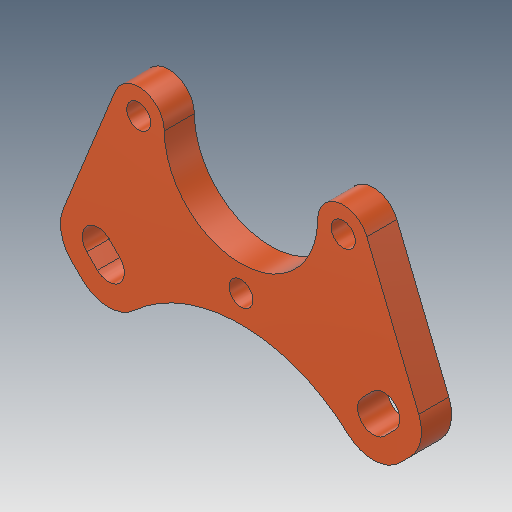
# Autodesk Inventor part: con_sensor_lod
Saved by Autodesk Inventor 2019.4 (Build 234330000, 330)
## iProperties
Created: 2018-07-20
Part Number: con_sensor_lod
Material: アルミニウム 6061
Document SubType Name: Modeling
Designer: student
Density: 2.7 g/cm^3
Appearance: 滑らか - 淡いオレンジ
Mass: 0.914676 g
Surface Area: 5.5303 cm^2
Volume: 0.338769 cm^3
Author: student
Autodesk Inventor part; units mm, degrees
ref_plane "YZ Plane" through (0, 0, 0) normal (1, 0, 0) x (0, 1, 0)
ref_plane "XZ Plane" through (0, 0, 0) normal (0, 1, 0) x (-1, 0, 0)
ref_plane "XY Plane" through (0, 0, 0) normal (0, 0, 1) x (1, 0, 0)
sketch "スケッチ1" plane through (0, 0, 0) normal (0, 0, 1) x (1, 0, 0)
  arc A0 (-5.1, 0) -> (0, -5.1) centre (0, 0) ccw
  arc A1 (-5.1, 0) -> (-8.3751, 0.6396) centre (-6.8, 0) ccw
  circle A2 centre (-6.8, 0) radius 0.8
  line L0 (0, 0) -> (-6.8, 0) construction
  line L1 (0, -5.1) -> (0, -6)
  line L2 (-10.573, -11.2802) -> (-11.2802, -10.573)
  line L3 (-11.8287, -7.8646) -> (-8.3751, 0.6396)
  line L4 (-10.2548, -9.5477) -> (-9.5477, -10.2548)
  line L5 (-8.7699, -8.0628) -> (-8.0628, -8.7699)
  arc A3 (-9.5477, -10.2548) -> (-8.0628, -8.7699) centre (-8.8053, -9.5124) ccw
  arc A4 (-8.7699, -8.0628) -> (-10.2548, -9.5477) centre (-9.5124, -8.8053) ccw
  circle A5 centre (-9.1588, -9.1588) radius 1.05 construction
  line L6 (-9.1588, -9.1588) -> (0, 0) construction
  arc A6 (-11.8287, -7.8646) -> (-11.2802, -10.573) centre (-9.5124, -8.8053) ccw
  arc A7 (-10.573, -11.2802) -> (-7.1206, -11.3595) centre (-8.8053, -9.5124) ccw
  arc A8 (0, -8.6) -> (-7.1206, -11.3595) centre (0, -19.1667) ccw
  line L7 (0, 0) -> (0, -5.1) construction
  circle A9 centre (0, -6.8) radius 0.8 construction
  arc A10 (0, -6) -> (0, -7.6) centre (0, -6.8) ccw
  line L8 (0, -7.6) -> (0, -8.6)
  circle A11 centre (-9.1588, -9.1588) radius 1 construction
  dimension "d0" = 10.2
  dimension "d3" = 6.8
  dimension "d4" = 1.6
  dimension "d6" = 2.1
  dimension "d9" = 1
  dimension "d11" = 2.5
  dimension "d12" = 8.6
  constraints: 18 end point, 18 point on circle, 12 tangent, 10 centre point, 4 concentric, 4 point on line, 3 equal radius, 3 vertical, 1 coincident, 1 horizontal, 1 perpendicular, 1 symmetric about line
  measures "d0" diameter of A0
  measures "d3" distance of L0.start L0.end
  measures "d4" diameter of A2
  measures "d6" diameter of A5
  measures "d9" distance of A4.centre A3.centre
  measures "d11" radius of A6
  measures "d12" distance from line of L0 L8.end
extrude "押し出し1" add sketch "スケッチ1" along normal blind 2
mirror "ミラー1" about plane through (0, -6, 0) normal (1, 0, 0) of "押し出し1"
